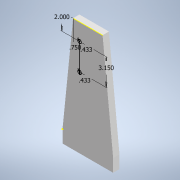
# Autodesk Inventor part: Gantry Panel
Saved by Autodesk Inventor 2022.3 (Build 263350000, 350)
## iProperties
Created: 2022-06-13
Part Number: Gantry Panel
Material: Generic
Document SubType Name: Modeling
Designer: Robert Nies
Density: 1 g/cm^3
Appearance: Default
Author: Robert Nies
Autodesk Inventor part; units mm, degrees
ref_plane "YZ Plane" through (0, 0, 0) normal (1, 0, 0) x (0, 1, 0)
ref_plane "XZ Plane" through (0, 0, 0) normal (0, 1, 0) x (-1, 0, 0)
ref_plane "XY Plane" through (0, 0, 0) normal (0, 0, 1) x (1, 0, 0)
sketch "Sketch1" plane through (0, 0, 0) normal (0, 0, 1) x (1, 0, 0)
  line L0 (0, 0) -> (152.4, 0)
  line L1 (152.4, 0) -> (152.4, -38.1)
  line L2 (152.4, -38.1) -> (0, -38.1)
  line L3 (0, -38.1) -> (0, 0)
  line L4 (0, 0) -> (31.75, 304.8)
  line L5 (31.75, 304.8) -> (120.65, 304.8)
  line L6 (120.65, 304.8) -> (152.4, 0)
  dimension "d0" = 152.4
  dimension "d1" = 38.1
  dimension "d2" = 88.9
  dimension "d3" = 31.75
  dimension "d4" = 304.8
  constraints: 14 end point, 2 horizontal, 2 parallel, 1 perpendicular
  measures "d0" distance of L1.end L2.end
  measures "d1" distance of L0.end L1.end
  measures "d2" distance of L4.end L5.end
  measures "d3" horizontal distance of L0.start L4.end
  measures "d4" vertical distance of L4.end L0.start
extrude "Extrusion1" add sketch "Sketch1" along normal blind 19.05
sketch "Sketch2" plane through (0, 0, 19.05) normal (0, 0, 1) x (1, 0, 0)
  circle A0 centre (82.55, 241.3) radius 5.5
  circle A1 centre (82.55, 161.3) radius 5.5
  line L0 (82.55, 241.3) -> (82.55, 161.3)
  line L1 (120.65, 304.8) -> (31.75, 304.8) projected
  point P0 (0, 0)
  dimension "d7" = 11
  dimension "d8" = 11
  dimension "d9" = 80
  dimension "d10" = 63.5
  dimension "d11" = 50.8
  constraints: 2 centre point, 2 end point, 1 vertical
  measures "d7" diameter of A0
  measures "d8" diameter of A1
  measures "d9" distance of L0.start L0.end
  measures "d10" distance from line of L1 L0.start
  measures "d11" horizontal distance of L1.end L0.start
extrude "Extrusion2" cut sketch "Sketch2" against normal blind 19.05
equation "\"d3\" = -0.5 * d2 + 0.5 * d0"
body "Solid1"
